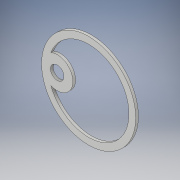
# Autodesk Inventor part: RO
Saved by Autodesk Inventor 2019 (Build 230136000, 136)
## iProperties
Created: 2019-10-19
Part Number: RO
Material: Generic
Document SubType Name: Modeling
Designer: Connor Duggan
Density: 1 g/cm^3
Appearance: Default
Author: Connor Duggan
Autodesk Inventor part; units mm, degrees
ref_plane "YZ Plane" through (0, 0, 0) normal (1, 0, 0) x (0, 1, 0)
ref_plane "XZ Plane" through (0, 0, 0) normal (0, 1, 0) x (-1, 0, 0)
ref_plane "XY Plane" through (0, 0, 0) normal (0, 0, 1) x (1, 0, 0)
sketch "Sketch1" plane through (0, 0, 0) normal (0, 0, 1) x (1, 0, 0)
  circle A0 centre (0, 0) radius 44.45
  line L0 (-44.45, 0) -> (-29.6672, 0) construction
  circle A1 centre (-29.6672, 0) radius 6.35
  arc A2 (-35.6191, -13.5238) -> (-35.6191, 13.5238) centre (0, 0) ccw
  arc A3 (-35.6191, -13.5238) -> (-35.6191, 13.5238) centre (-29.6672, 0) ccw
  dimension "d0" = 88.9
  dimension "d6" = 14.7828
  dimension "d7" = 12.7
  dimension "d8" = 76.2
  constraints: 4 coincident, 4 point on circle, 3 centre point, 2 end point, 1 horizontal, 1 horizontal alignment, 2 other
  measures "d6" distance of L0.start L0.end
  measures "d7" diameter of A1
  measures "d8" diameter of A2
extrude "Extrusion3" add sketch "Sketch1" along normal blind 2.54
body "Solid2"
